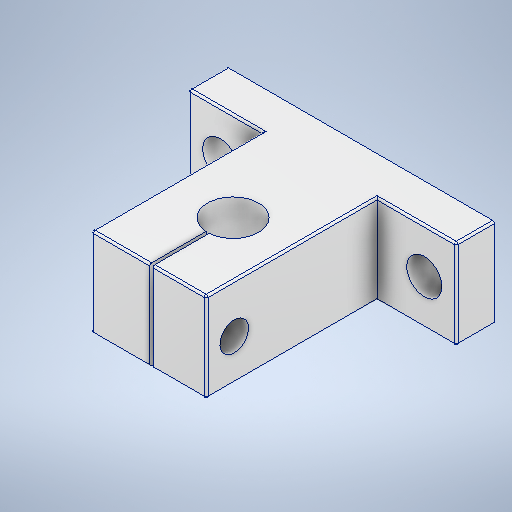
# Autodesk Inventor part: SK8_LinearShaftSupport
Saved by Autodesk Inventor 2025.2 (Build 292293000, 293)
## iProperties
Created: 2022-05-28
Part Number: SK8_LinearShaftSupport
Material: Aluminum 6061
Document SubType Name: Modeling
Designer: mdff2
Density: 2.7 g/cm^3
Appearance: Aluminum - Flat
Author: mdff2
Autodesk Inventor part; units mm, degrees
ref_plane "YZ Plane" through (0, 0, 0) normal (1, 0, 0) x (0, 1, 0)
ref_plane "XZ Plane" through (0, 0, 0) normal (0, 1, 0) x (-1, 0, 0)
ref_plane "XY Plane" through (0, 0, 0) normal (0, 0, 1) x (1, 0, 0)
sketch "Boceto1" plane through (0, 0, 0) normal (0, 0, 1) x (1, 0, 0)
  line L0 (-19.271, 0) -> (-1.6402, 0)
  circle A0 centre (-16, 0) radius 2.75
  circle A1 centre (16, 0) radius 2.75
  line L1 (21, -7) -> (-21, -7)
  line L2 (-21, -7) -> (-21, 7)
  line L3 (-21, 7) -> (21, 7)
  line L4 (21, 7) -> (21, -7)
  line L5 (21, -7) -> (-21, 7) construction
  line L6 (-21, -7) -> (21, 7) construction
  point P0 (0, 0)
  point P1 (0, 0)
  dimension "d0" = 5.5
  dimension "d1" = 5.5
  dimension "d2" = 16
  dimension "d3" = 32
  dimension "d4" = 14
  dimension "d5" = 42
  constraints: 14 end point, 2 centre point, 2 horizontal, 2 midpoint, 2 parallel, 2 point on line, 1 coincident, 1 perpendicular
  measures "d0" diameter of A0
  measures "d1" diameter of A1
  measures "d2" distance of point (0, 0) A0.centre
  measures "d3" distance of A0.centre A1.centre
  measures "d4" distance of L1.end L2.end
  measures "d5" distance of L1.start L1.end
extrude "Extrusión1" add sketch "Boceto1" along normal blind 6
sketch "Boceto2" plane through (0, 0, 6) normal (0, 0, 1) x (1, 0, 0)
  point P0 (0, 0)
sketch "Boceto3" plane through (0, 0, 0) normal (0, 1, 0) x (-1, 0, 0)
  line L0 (-21, 0) -> (21, 0) projected
  line L1 (-8.586, 32.8) -> (-8.586, 0)
  line L2 (-8.586, 0) -> (9.414, 0)
  line L3 (9.414, 0) -> (9.414, 32.8)
  arc A0 (-0.25, 23.9922) -> (0.25, 23.9922) centre (0, 20) ccw
  line L4 (0.25, 36.8) -> (-0.25, 36.8)
  line L5 (-0.25, 32.8) -> (-0.25, 22.8)
  line L6 (-0.25, 22.8) -> (0.25, 22.8)
  line L7 (0.25, 22.8) -> (0.25, 32.8)
  line L8 (0.25, 36.8) -> (-0.25, 22.8) construction
  line L9 (-0.25, 36.8) -> (0.25, 22.8) construction
  line L10 (9.414, 32.8) -> (0.25, 32.8)
  line L11 (-0.25, 32.8) -> (-8.586, 32.8)
  point P0 (0, 0)
  dimension "d8" = 32.8
  dimension "d9" = 8
  dimension "d10" = 20
  dimension "d12" = 18
  dimension "d13" = 0.5
  dimension "d14" = 14
  constraints: 22 end point, 5 parallel, 3 horizontal, 3 perpendicular, 3 point on line, 2 point on circle, 1 centre point
  measures "d8" distance of L2.end L3.end
  measures "d9" diameter of A0
  measures "d10" distance from line of L0 A0.centre
  measures "d12" distance of L3.end L1.start
  measures "d13" distance of L4.start L4.end
  measures "d14" distance of L6.end L4.start
extrude "Extrusión2" add sketch "Boceto3" against normal mid plane 14 contours L1 L11 L5 A0 L7 L10 L3 L0
fillet "Empalme1" radius 0.3 20 edges at (-4.832, -7, 32.8) (4.418, -7, 32.8) (-15.207, -7, 6) (14.793, -7, 6) (-21, 0, 6) (-21, 7, 3) (-21, -7, 3) (21, -7, 3) (21, 7, 3) (14.793, 7, 6) (21, 0, 6) (-15.207, 7, 6) (8.586, 0, 32.8) (-9.414, 0, 32.8) (8.586, 7, 19.4) (-9.414, 7, 19.4) (8.586, -7, 19.4) (-9.414, -7, 19.4) (-4.832, 7, 32.8) (4.418, 7, 32.8)
sketch "Boceto5" plane through (0, 0, 0) normal (1, 0, 0) x (0, 1, 0)
  circle A0 centre (-0.6204, 28.4) radius 2.25
  line L0 (6.7, 0) -> (-6.7, 0) projected
  point P0 (0, 0)
  dimension "d18" = 4.5
  dimension "d19" = 28.4
  constraints: 1 centre point
  measures "d18" diameter of A0
  measures "d19" distance from line of L0 A0.centre
extrude "Extrusión3" cut sketch "Boceto5" along normal mid plane 20
